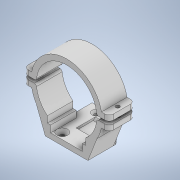
# Autodesk Inventor part: motor holder
Saved by Autodesk Inventor 2020 (Build 240168000, 168)
## iProperties
Created: 2026-07-07
Part Number: motor holder
Material: Generic
Document SubType Name: Modeling
Designer: drago
Density: 1 g/cm^3
Appearance: Default
Author: drago
Autodesk Inventor part; units mm, degrees
ref_plane "YZ Plane" through (0, 0, 0) normal (1, 0, 0) x (0, 1, 0)
ref_plane "XZ Plane" through (0, 0, 0) normal (0, 1, 0) x (-1, 0, 0)
ref_plane "XY Plane" through (0, 0, 0) normal (0, 0, 1) x (1, 0, 0)
sketch "Sketch1" plane through (0, 0, 0) normal (0, 0, 1) x (1, 0, 0)
  line L0 (-7.5, -12.0578) -> (-7.5, -17.2)
  line L1 (-7.5, -17.2) -> (7.5, -17.2)
  line L2 (7.5, -17.2) -> (7.5, -12.0578)
  arc A0 (7.5, -12.0578) -> (-7.5, -12.0578) centre (0, 0) ccw
  line L3 (-10, -13.375) -> (-10, -19.7)
  line L4 (-10, -19.7) -> (10, -19.7)
  line L5 (10, -19.7) -> (10, -13.375)
  arc A1 (10, -13.375) -> (-10, -13.375) centre (0, 0) ccw
  dimension "d1" = 2.5
  constraints: 12 end point, 4 point on circle, 2 centre point, 3 other
  measures "d1" radial gap between concentric circles of A0 A1
extrude "Extrusion1" add sketch "Sketch1" along normal blind 12
sketch "Sketch2" plane through (-10, -19.7, 0) normal (0, -1, 0) x (1, 0, 0)
  line L0 (0, 0) -> (20, 0) projected
  line L1 (20, 0) -> (0, 0)
  line L2 (0, 0) -> (0, -10)
  line L3 (0, -10) -> (20, -10)
  line L4 (20, -10) -> (20, 0)
  point P0 (10, 0)
  dimension "d4" = 10
  constraints: 8 end point, 2 parallel, 1 horizontal, 1 perpendicular
  measures "d4" distance of L2.end L1.end
extrude "Extrusion2" add sketch "Sketch2" against normal blind 2.5
sketch "Sketch3" plane through (-10, -19.7, 12) normal (0, -1, 0) x (1, 0, 0)
  line L0 (0, -22) -> (0, -12) projected
  line L1 (0, -22) -> (12, -22)
  line L2 (20, -22) -> (0, -22) projected
  line L3 (12, -22) -> (16.5, -22)
  line L4 (16.5, -22) -> (16.5, -11.1)
  line L5 (16.5, -11.1) -> (12, -11.1)
  line L6 (12, -11.1) -> (12, -22)
  circle A0 centre (16.5, -11.1) radius 1.5
  circle A1 centre (16.5, -11.1) radius 4
  line L7 (12, -22) -> (19.4603, -13.79)
  line L8 (20, -22) -> (20, -13.0365)
  line L9 (20, -12) -> (20, -22) projected
  point P0 (10, -12)
  dimension "d7" = 12
  dimension "d8" = 4.5
  dimension "d9" = 10.9
  dimension "d10" = 3
  dimension "d11" = 8
  constraints: 14 end point, 2 centre point, 2 coincident, 2 parallel, 2 point on circle, 2 point on line, 1 horizontal, 1 perpendicular, 1 tangent
  measures "d7" distance of L0.start L1.end
  measures "d8" distance of L5.end L4.end
  measures "d9" distance of L4.end L3.end
  measures "d10" diameter of A0
  measures "d11" diameter of A1
extrude "Extrusion3" cut sketch "Sketch3" against normal blind 2.5 contours L2 L4 L7 A1 L8 | L2 L7 L4
sketch "Sketch4" plane through (-10, -19.7, 12) normal (0, -1, 0) x (1, 0, 0)
  circle A0 centre (5, -19) radius 1
  circle A1 centre (11, -19) radius 1
  point P0 (10, -12)
  point P1 (0, -22)
  constraints: 2 centre point
extrude "Extrusion4" cut sketch "Sketch4" against normal blind 2.5
sketch "Sketch5" plane through (-10, -19.7, 12) normal (0, -1, 0) x (1, 0, 0)
  circle A0 centre (5, -19) radius 1 projected
  circle A1 centre (5, -3) radius 1
  point P0 (10, -12)
  constraints: 1 centre point
extrude "Extrusion5" cut sketch "Sketch5" against normal blind 2.5 contours A1
chamfer "Chamfer1" distance 1.5 angle 45 1 edges at (-6, -17.2, 9)
sketch "Sketch6" plane through (0, 0, 0) normal (0, 0, -1) x (-1, 0, 0)
  line L0 (-20, -3.25) -> (20, -3.25)
  line L1 (20, -3.25) -> (20, 3.25)
  line L2 (20, 3.25) -> (-20, 3.25)
  line L3 (-20, 3.25) -> (-20, -3.25)
  line L4 (20, -0.75) -> (-20, -0.75)
  line L5 (-20, -0.75) -> (-20, 0.75)
  line L6 (-20, 0.75) -> (20, 0.75)
  line L7 (20, 0.75) -> (20, -0.75)
  arc A0 (10, -13.375) -> (-10, -13.375) centre (0, 0) ccw projected
  point P0 (16.3807, 3.25)
  point P1 (16.6832, 0.75)
  point P2 (16.6832, -0.75)
  point P3 (16.3807, -3.25)
  point P4 (-16.6832, 0.75)
  point P5 (-16.3807, 3.25)
  point P6 (-16.3807, -3.25)
  point P7 (-16.6832, -0.75)
  constraints: 16 end point, 4 parallel, 2 horizontal, 2 perpendicular, 1 point on line
extrude "Extrusion6" add sketch "Sketch6" against normal up to surface (12 mm away) contours L3 L4 A0 L0 | A0 L4 L1 L0 | L3 L2 A0 L6 | A0 L2 L1 L6
extrude "Extrusion7" cut sketch "Sketch6" against normal blind 20 contours A0 L6 L4
sketch "Sketch7" plane through (16.3807, 3.25, 0) normal (0, 1, 0) x (1, 0, 0)
  line L0 (3.6193, 0) -> (3.6193, -12) projected
  line L1 (-36.3807, 0) -> (-36.3807, -12) projected
  circle A0 centre (-34.3807, -6) radius 0.9
  circle A1 centre (1.6193, -6) radius 0.9
  point P0 (-16.3807, 0)
  dimension "d37" = 1.8
  constraints: 2 centre point
  measures "d37" diameter of A0
extrude "Extrusion8" cut sketch "Sketch7" against normal blind 20
fillet "Fillet1" radius 2 8 edges at (20, -2, 0) (20, 2, 0) (20, -2, 12) (20, 2, 12) (-20, -2, 0) (-20, 2, 0) (-20, 2, 12) (-20, -2, 12)
fillet "Fillet2" radius 1 4 edges at (14.1802, -0.75, 6) (-14.1802, -0.75, 6) (14.1802, 0.75, 6) (-14.1802, 0.75, 6)
fillet "Fillet3" radius 1 2 edges at (7.5, -12.0578, 6) (-7.5, -12.0578, 6)
chamfer "Chamfer2" distance 1 angle 45 2 edges at (-6, -17.2, -7) (0, -17.2, -7)
sketch "Sketch8" plane through (-7.5, -17.2, 12) normal (0, 1, 0) x (1, 0, 0)
  line L0 (0, 12) -> (15, 12)
  line L1 (11, 8) -> (4, 8)
  line L2 (4, 8) -> (4, 16)
  line L3 (4, 16) -> (11, 16)
  line L4 (11, 16) -> (11, 8)
  line L5 (11, 8) -> (4, 16) construction
  line L6 (4, 8) -> (11, 16) construction
  point P0 (7.5, 12)
  dimension "d47" = 7
  dimension "d48" = 8
  constraints: 14 end point, 2 horizontal, 2 midpoint, 2 parallel, 1 perpendicular
  measures "d47" distance of L2.end L3.end
  measures "d48" distance of L1.end L2.end
extrude "Extrusion9" cut sketch "Sketch8" against normal blind 1
chamfer "Chamfer3" distance 1 angle 45 1 edges at (0, -17.2, -4)
sketch "Sketch9" plane through (0, 0, 0) normal (0, 0, -1) x (-1, 0, 0)
  line L0 (0, 0) -> (9, 0)
  line L1 (9, 0) -> (9, -14)
  line L2 (9, -14) -> (0, -14)
  line L3 (0, -14) -> (0, 0)
  line L4 (0, 0) -> (-9, 0)
  line L5 (-9, 0) -> (-9, -14)
  line L6 (-9, -14) -> (0, -14)
  line L7 (0, -14) -> (0, 0)
  constraints: 16 end point, 4 parallel, 2 horizontal, 2 perpendicular, 1 point on line
extrude "Extrusion10" cut sketch "Sketch9" against normal blind 20
sketch "Sketch10" plane through (0, 0, 0) normal (0, 0, -1) x (-1, 0, 0)
  arc A0 (-16.3807, -3.25) -> (-10, -13.375) centre (0, 0) ccw projected
  line L0 (10, -19.7) -> (-10, -19.7) projected
  line L1 (-16.3807, -3.25) -> (-10, -19.7)
  line L2 (10, -13.375) -> (10, -19.7) projected
  line L3 (16.3807, -3.25) -> (18, -3.25) projected
  line L4 (10, -19.7) -> (16.3807, -3.25)
  line L5 (-10, -17.2) -> (-10, -13.375) projected
  line L6 (-10, -19.7) -> (-10, -17.2) projected
  line L7 (10, -19.7) -> (10, -17.2) projected
  arc A1 (10, -13.375) -> (16.3807, -3.25) centre (0, 0) ccw projected
  point P0 (-14.2877, -8.6458)
  point P1 (14.2877, -8.6458)
  constraints: 4 end point
extrude "Extrusion11" add sketch "Sketch10" against normal up to surface (12 mm away) contours A0 L5 L6 L1 | A1 L4 L2
body "Solid1"
